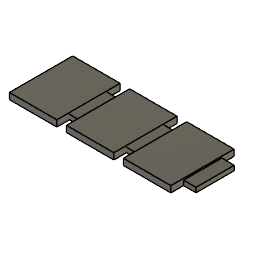
solarpanels (Autodesk Fusion 360 design; units mm, degrees)
Autodesk Fusion 360 part; units mm, degrees
sketch "Sketch1" plane through (0, 0, 0) normal (0, 0, 1) x (1, 0, 0)
  line L0 (-63.5, 25.4) -> (-44.45, 25.4)
  line L1 (-44.45, 25.4) -> (-44.45, 0)
  line L2 (-44.45, 0) -> (-63.5, 0)
  line L3 (-63.5, 0) -> (-63.5, 25.4)
  line L4 (-44.45, 20.2856) -> (-40.64, 20.2856)
  line L5 (-40.64, 20.2856) -> (-40.64, 5.0456)
  line L6 (-40.64, 5.0456) -> (-44.45, 5.0456)
  line L7 (-44.45, 5.0456) -> (-44.45, 20.2856)
  line L8 (-40.64, 0) -> (-21.59, 0)
  line L9 (-21.59, 0) -> (-21.59, 25.4)
  line L10 (-21.59, 25.4) -> (-40.64, 25.4)
  line L11 (-40.64, 25.4) -> (-40.64, 0)
  line L12 (-21.59, 5.0849) -> (-17.78, 5.0849)
  line L13 (-17.78, 5.0849) -> (-17.78, 20.32)
  line L14 (-17.78, 20.32) -> (-21.59, 20.32)
  line L15 (-21.59, 20.32) -> (-21.59, 5.0849)
  line L16 (-17.78, 25.4) -> (1.27, 25.4)
  line L17 (1.27, 25.4) -> (1.27, 0)
  line L18 (1.27, 0) -> (-17.78, 0)
  line L19 (-17.78, 0) -> (-17.78, 25.4)
  line L20 (1.27, 20.2099) -> (5.08, 20.2099)
  line L21 (5.08, 20.2099) -> (5.08, 4.9699)
  line L22 (5.08, 4.9699) -> (1.27, 4.9699)
  line L23 (1.27, 4.9699) -> (1.27, 20.2099)
  dimension "d1" = 19.05
  dimension "d2" = 25.4
  dimension "d3" = 15.24
  dimension "d4" = 19.05
  dimension "d5" = 19.05
  dimension "d6" = 3.81
  dimension "d7" = 15.24
  constraint horizontal L0
  constraint vertical L1
  constraint horizontal L2
  constraint vertical L3
  constraint horizontal L4
  constraint vertical L5
  constraint horizontal L6
  constraint vertical L7
  constraint coincident L1 L4.start
  constraint horizontal L8
  constraint vertical L9
  constraint horizontal L10
  constraint vertical L11
  constraint horizontal L12
  constraint vertical L13
  constraint horizontal L14
  constraint vertical L15
  constraint coincident L9 L12.start
  constraint horizontal L16
  constraint vertical L17
  constraint horizontal L18
  constraint vertical L19
  constraint horizontal L20
  constraint vertical L21
  constraint horizontal L22
  constraint vertical L23
  constraint coincident L17 L20.start
  measures "d1" distance of L0.start L0.end
  measures "d2" distance of L0.start L2.end
  measures "d3" distance of L4.start L6.end
  measures "d4" distance of L8.start L8.end
  measures "d5" distance of L16.start L16.end
  measures "d6" distance of L20.start L20.end
  measures "d7" distance of L20.start L22.end
extrude "Extrude1" add sketch "Sketch1" along normal blind 2.54 contours L0 L1 L2 L3 L7 | L5 L8 L9 L10 L11 L15 | L13 L16 L17 L18 L19 L23 makes body 1 at (-11.43, 16.9333, 0) makes body 2 at (-34.29, 16.9333, 0) makes body 3 at (-57.15, 8.4667, 0)
sketch "Sketch2" plane through (0, 0, 0) normal (0, 0, 1) x (1, 0, 0)
  line L0 (-50.8, 20.32) -> (-10.16, 20.32)
  line L1 (-10.16, 20.32) -> (-10.16, 5.08)
  line L2 (-10.16, 5.08) -> (-50.8, 5.08)
  line L3 (-50.8, 5.08) -> (-50.8, 20.32)
  constraint horizontal L0
  constraint vertical L1
  constraint horizontal L2
  constraint vertical L3
extrude "Extrude2" add sketch "Sketch2" along normal blind 1.905 separate body makes body 4
sketch "Sketch3" plane through (1.27, 0, 0) normal (1, 0, 0) x (0, 1, 0)
  line L0 (0, 0) -> (25.4, 0)
  line L1 (25.4, 0) -> (25.4, 2.54)
  line L2 (25.4, 2.54) -> (0, 2.54)
  line L3 (0, 2.54) -> (0, 0)
  line L4 (5.08, 0) -> (20.4638, 0)
  line L5 (20.4638, 0) -> (20.4638, 1.2766)
  line L6 (20.4638, 1.2766) -> (5.08, 1.2766)
  line L7 (5.08, 1.2766) -> (5.08, 0)
  constraint horizontal L4
  constraint vertical L5
  constraint horizontal L6
  constraint vertical L7
  constraint coincident L0 L4.start
extrude "Extrude3" add sketch "Sketch3" along normal blind 5.0038 contours L0 L4 L5 L6 L7 bodies 1
extrude "Extrude4" add 1 faces at (2.9379, 15.3358, 1.2766) along direction (0, 0, 1) blind 0.635 on bodies 1 bodies 1
